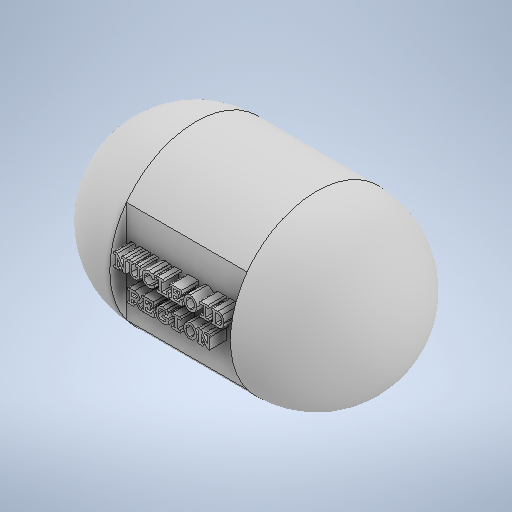
# Autodesk Inventor part: Nucleoid Region
Saved by Autodesk Inventor 2025 (Build 290162000, 162)
## iProperties
Created: 2024-09-07
Part Number: Nucleoid Region
Material: Generic
Document SubType Name: Modeling
Designer: kellst1
Density: 1 g/cm^3
Appearance: Default
Author: kellst1
Autodesk Inventor part; units mm, degrees
ref_plane "YZ Plane" through (0, 0, 0) normal (1, 0, 0) x (0, 1, 0)
ref_plane "XZ Plane" through (0, 0, 0) normal (0, 1, 0) x (-1, 0, 0)
sketch "Sketch2" plane through (0, 0, 0) normal (1, 0, 0) x (0, 1, 0)
  circle A0 centre (0, 0) radius 25
  dimension "d0" = 50
  constraints: 1 centre point, 1 coincident
  measures "d0" diameter of A0
extrude "Extrusion1" add sketch "Sketch2" along normal blind 35
sketch "Sketch3" plane through (35, 0, 0) normal (1, 0, 0) x (0, 0, -1)
  arc A0 (25, 0) -> (-25, 0) centre (0, 0) ccw
  line L0 (-25, 0) -> (25, 0)
  constraints: 2 end point, 2 point on circle, 1 centre point, 1 coincident, 1 horizontal
revolve "Revolution1" add sketch "Sketch3" angle 180 about axis through (35, 0, 25) along (0, 0, -1)
sketch "Sketch4" plane through (0, 0, 0) normal (-1, 0, 0) x (0, 0, 1)
  circle A0 centre (0, 0) radius 25 projected
  line L0 (20.1665, 14.7754) -> (33.009, 14.7754)
  line L1 (33.009, 14.7754) -> (33.009, -19.9353)
  line L2 (33.009, -19.9353) -> (20.1665, -19.9353)
  line L3 (20.1665, -19.9353) -> (20.1665, 14.7754)
  point P0 (20.1665, -14.7754)
  constraints: 8 end point, 2 parallel, 1 horizontal, 1 perpendicular, 2 other
extrude "Extrusion2" cut sketch "Sketch4" against normal blind 35 contours A0 L3 picked at (21.0481, -3.4098)
ref_plane "Work Plane1" through (17.5, 0, 0) normal (-1, 0, 0) x (0, 0, 1)
mirror "Mirror1" about plane through (17.5, 0, 0) normal (-1, 0, 0) of "Revolution1"
sketch "Sketch8" plane through (35, -14.7754, 20.1665) normal (0, 0, 1) x (1, 0, 0)
  line L0 (-34.9965, 29.6893) -> (-0.1735, 29.6893) construction
  line L1 (-0.1735, 29.6893) -> (-0.1735, 0.1878) construction
  line L2 (-0.1735, 0.1878) -> (-34.9965, 0.1878) construction
  line L3 (-34.9965, 0.1878) -> (-34.9965, 29.6893) construction
  line L4 (-32.6139, 19.1334) -> (-32.6139, 17.0905)
  line L5 (-32.6139, 17.0905) -> (-32.3712, 17.0905)
  spline S0 degree 2 poles (-32.3712, 17.0905) (-32.1172, 17.0905) (-31.908, 16.9037) (-31.908, 16.7506) knots 0 0 0 1 2 2 2
  spline S1 degree 2 poles (-31.908, 16.7506) (-31.908, 16.5975) (-32.1172, 16.4145) (-32.3712, 16.4145) knots 0 0 0 1 2 2 2
  line L6 (-32.3712, 16.4145) -> (-33.2899, 16.4145)
  spline S2 degree 2 poles (-33.2899, 16.4145) (-33.5439, 16.4145) (-33.753, 16.6012) (-33.753, 16.7543) knots 0 0 0 1 2 2 2
  spline S3 degree 2 poles (-33.753, 16.7543) (-33.753, 16.9075) (-33.5439, 17.0905) (-33.2899, 17.0905) knots 0 0 0 1 2 2 2
  line L7 (-33.2899, 17.0905) -> (-33.2899, 19.7385)
  line L8 (-33.2899, 19.7385) -> (-33.3945, 19.7385)
  spline S4 degree 2 poles (-33.3945, 19.7385) (-33.6485, 19.7385) (-33.8576, 19.9252) (-33.8576, 20.0783) knots 0 0 0 1 2 2 2
  spline S5 degree 2 poles (-33.8576, 20.0783) (-33.8576, 20.2277) (-33.6485, 20.4145) (-33.3945, 20.4145) knots 0 0 0 1 2 2 2
  line L9 (-33.3945, 20.4145) -> (-32.6177, 20.4107)
  line L10 (-32.6177, 20.4107) -> (-30.881, 17.6992)
  line L11 (-30.881, 17.6992) -> (-30.881, 19.7385)
  line L12 (-30.881, 19.7385) -> (-31.1237, 19.7385)
  spline S6 degree 2 poles (-31.1237, 19.7385) (-31.3777, 19.7385) (-31.5868, 19.9252) (-31.5868, 20.0783) knots 0 0 0 1 2 2 2
  spline S7 degree 2 poles (-31.5868, 20.0783) (-31.5868, 20.2277) (-31.3777, 20.4145) (-31.1237, 20.4145) knots 0 0 0 1 2 2 2
  line L13 (-31.1237, 20.4145) -> (-30.205, 20.4107)
  spline S8 degree 2 poles (-30.205, 20.4107) (-29.951, 20.4107) (-29.7418, 20.2277) (-29.7418, 20.0746) knots 0 0 0 1 2 2 2
  spline S9 degree 2 poles (-29.7418, 20.0746) (-29.7418, 19.9215) (-29.951, 19.7347) (-30.205, 19.7347) knots 0 0 0 1 2 2 2
  line L14 (-30.205, 19.7347) -> (-30.205, 16.4145)
  line L15 (-30.205, 16.4145) -> (-30.8698, 16.4145)
  line L16 (-30.8698, 16.4145) -> (-32.6139, 19.1334)
  line L17 (-26.1713, 19.7347) -> (-26.1713, 17.8188)
  spline S10 degree 2 poles (-26.1713, 17.8188) (-26.1713, 17.195) (-27.0714, 16.3174) (-27.7026, 16.3174) knots 0 0 0 1 2 2 2
  spline S11 degree 2 poles (-27.7026, 16.3174) (-28.0164, 16.3174) (-28.5654, 16.5377) (-29.0061, 16.9672) (-29.2488, 17.4303) (-29.2488, 17.8188) knots 0 0 0 1 2 3 4 4 4
  line L18 (-29.2488, 17.8188) -> (-29.2488, 19.7347)
  spline S12 degree 2 poles (-29.2488, 19.7347) (-29.5028, 19.7347) (-29.712, 19.9215) (-29.712, 20.0746) knots 0 0 0 1 2 2 2
  spline S13 degree 2 poles (-29.712, 20.0746) (-29.712, 20.2277) (-29.5028, 20.4107) (-29.2488, 20.4107) knots 0 0 0 1 2 2 2
  line L19 (-29.2488, 20.4107) -> (-28.3301, 20.4145)
  spline S14 degree 2 poles (-28.3301, 20.4145) (-28.1097, 20.4145) (-27.9006, 20.2277) (-27.9006, 20.0783) knots 0 0 0 1 2 2 2
  spline S15 degree 2 poles (-27.9006, 20.0783) (-27.9006, 19.9252) (-28.1097, 19.7385) (-28.3301, 19.7385) knots 0 0 0 1 2 2 2
  line L20 (-28.3301, 19.7385) -> (-28.5728, 19.7385)
  line L21 (-28.5728, 19.7385) -> (-28.5728, 17.7627)
  spline S16 degree 2 poles (-28.5728, 17.7627) (-28.5728, 17.4602) (-28.0686, 16.9934) (-27.7138, 16.9934) knots 0 0 0 1 2 2 2
  spline S17 degree 2 poles (-27.7138, 16.9934) (-27.4748, 16.9934) (-27.0602, 17.2174) (-26.9295, 17.4341) knots 0 0 0 1 2 2 2
  spline S18 degree 2 poles (-26.9295, 17.4341) (-26.8474, 17.5685) (-26.8474, 17.7627) knots 0 0 0 1 1 1
  line L22 (-26.8474, 17.7627) -> (-26.8474, 19.7385)
  line L23 (-26.8474, 19.7385) -> (-27.0901, 19.7385)
  spline S19 degree 2 poles (-27.0901, 19.7385) (-27.3105, 19.7385) (-27.5196, 19.9252) (-27.5196, 20.0783) knots 0 0 0 1 2 2 2
  spline S20 degree 2 poles (-27.5196, 20.0783) (-27.5196, 20.2277) (-27.3105, 20.4145) (-27.0901, 20.4145) knots 0 0 0 1 2 2 2
  line L24 (-27.0901, 20.4145) -> (-26.1713, 20.4107)
  spline S21 degree 2 poles (-26.1713, 20.4107) (-25.9174, 20.4107) (-25.7082, 20.2277) (-25.7082, 20.0746) knots 0 0 0 1 2 2 2
  spline S22 degree 2 poles (-25.7082, 20.0746) (-25.7082, 19.9215) (-25.9174, 19.7347) (-26.1713, 19.7347) knots 0 0 0 1 2 2 2
  spline S23 degree 2 poles (-22.6046, 20.2389) (-22.5411, 20.3248) (-22.3917, 20.4107) (-22.3058, 20.4107) knots 0 0 0 1 2 2 2
  spline S24 degree 2 poles (-22.3058, 20.4107) (-22.1564, 20.4107) (-21.9697, 20.2053) (-21.9697, 19.9625) knots 0 0 0 1 2 2 2
  line L25 (-21.9697, 19.9625) -> (-21.9697, 19.3874)
  spline S25 degree 2 poles (-21.9697, 19.3874) (-21.9697, 19.1446) (-22.1564, 18.9355) (-22.3058, 18.9355) knots 0 0 0 1 2 2 2
  spline S26 degree 2 poles (-22.3058, 18.9355) (-22.4403, 18.9355) (-22.5224, 19.0102) knots 0 0 0 1 1 1
  spline S27 degree 2 poles (-22.5224, 19.0102) (-22.6046, 19.0886) (-22.6457, 19.294) knots 0 0 0 1 1 1
  spline S28 degree 2 poles (-22.6457, 19.294) (-22.6681, 19.4322) (-22.739, 19.5106) knots 0 0 0 1 1 1
  spline S29 degree 2 poles (-22.739, 19.5106) (-22.8735, 19.6563) (-23.359, 19.8356) (-23.6018, 19.8356) knots 0 0 0 1 2 2 2
  spline S30 degree 2 poles (-23.6018, 19.8356) (-23.9043, 19.8356) (-24.4122, 19.5704) (-24.8007, 18.9803) (-24.8007, 18.5695) knots 0 0 0 1 2 3 3 3
  line L26 (-24.8007, 18.5695) -> (-24.8007, 18.1325)
  spline S31 degree 2 poles (-24.8007, 18.1325) (-24.8007, 17.647) (-24.0911, 16.9934) (-23.4636, 16.9934) knots 0 0 0 1 2 2 2
  spline S32 degree 2 poles (-23.4636, 16.9934) (-23.0864, 16.9934) (-22.8287, 17.0942) knots 0 0 0 1 1 1
  spline S33 degree 2 poles (-22.8287, 17.0942) (-22.6756, 17.154) (-22.5037, 17.3295) knots 0 0 0 1 1 1
  spline S34 degree 2 poles (-22.5037, 17.3295) (-22.3992, 17.4341) (-22.2797, 17.4976) (-22.205, 17.4976) knots 0 0 0 1 2 2 2
  spline S35 degree 2 poles (-22.205, 17.4976) (-22.0705, 17.4976) (-21.8651, 17.2921) (-21.8651, 17.154) knots 0 0 0 1 2 2 2
  spline S36 degree 2 poles (-21.8651, 17.154) (-21.8651, 17.0158) (-22.0033, 16.8589) knots 0 0 0 1 1 1
  spline S37 degree 2 poles (-22.0033, 16.8589) (-22.205, 16.6273) (-22.5224, 16.4966) knots 0 0 0 1 1 1
  spline S38 degree 2 poles (-22.5224, 16.4966) (-22.9445, 16.3174) (-23.4599, 16.3174) knots 0 0 0 1 1 1
  spline S39 degree 2 poles (-23.4599, 16.3174) (-24.0612, 16.3174) (-24.5392, 16.5639) knots 0 0 0 1 1 1
  spline S40 degree 2 poles (-24.5392, 16.5639) (-24.9314, 16.7618) (-25.4767, 17.6171) (-25.4767, 18.1213) knots 0 0 0 1 2 2 2
  line L27 (-25.4767, 18.1213) -> (-25.4767, 18.5769)
  spline S41 degree 2 poles (-25.4767, 18.5769) (-25.4767, 19.1035) (-24.9874, 20.0186) (-24.1172, 20.5116) (-23.6279, 20.5116) knots 0 0 0 1 2 3 3 3
  spline S42 degree 2 poles (-23.6279, 20.5116) (-23.3366, 20.5116) (-22.8249, 20.3771) (-22.6046, 20.2389) knots 0 0 0 1 2 2 2
  line L28 (-19.8931, 19.7347) -> (-19.8931, 17.0905)
  line L29 (-19.8931, 17.0905) -> (-18.4365, 17.0905)
  line L30 (-18.4365, 17.0905) -> (-18.4365, 17.7291)
  spline S43 degree 2 poles (-18.4365, 17.7291) (-18.4365, 17.9831) (-18.2498, 18.1922) (-18.0967, 18.1922) knots 0 0 0 1 2 2 2
  spline S44 degree 2 poles (-18.0967, 18.1922) (-17.9435, 18.1922) (-17.7605, 17.9831) (-17.7605, 17.7291) knots 0 0 0 1 2 2 2
  line L31 (-17.7605, 17.7291) -> (-17.7605, 16.4145)
  line L32 (-17.7605, 16.4145) -> (-20.9613, 16.4145)
  spline S45 degree 2 poles (-20.9613, 16.4145) (-21.2152, 16.4145) (-21.4244, 16.6012) (-21.4244, 16.7543) knots 0 0 0 1 2 2 2
  spline S46 degree 2 poles (-21.4244, 16.7543) (-21.4244, 16.9075) (-21.2152, 17.0905) (-20.9613, 17.0905) knots 0 0 0 1 2 2 2
  line L33 (-20.9613, 17.0905) -> (-20.5691, 17.0905)
  line L34 (-20.5691, 17.0905) -> (-20.5691, 19.7385)
  line L35 (-20.5691, 19.7385) -> (-20.9613, 19.7385)
  spline S47 degree 2 poles (-20.9613, 19.7385) (-21.2152, 19.7385) (-21.4244, 19.9252) (-21.4244, 20.0783) knots 0 0 0 1 2 2 2
  spline S48 degree 2 poles (-21.4244, 20.0783) (-21.4244, 20.2277) (-21.2152, 20.4145) (-20.9613, 20.4145) knots 0 0 0 1 2 2 2
  line L36 (-20.9613, 20.4145) -> (-19.4972, 20.4107)
  spline S49 degree 2 poles (-19.4972, 20.4107) (-19.2432, 20.4107) (-19.0341, 20.2277) (-19.0341, 20.0746) knots 0 0 0 1 2 2 2
  spline S50 degree 2 poles (-19.0341, 20.0746) (-19.0341, 19.9215) (-19.2432, 19.7347) (-19.4972, 19.7347) knots 0 0 0 1 2 2 2
  line L37 (-19.4972, 19.7347) -> (-19.8931, 19.7347)
  line L38 (-16.2516, 18.0839) -> (-16.2516, 17.0905)
  line L39 (-16.2516, 17.0905) -> (-14.5262, 17.0905)
  line L40 (-14.5262, 17.0905) -> (-14.5262, 17.4565)
  spline S51 degree 2 poles (-14.5262, 17.4565) (-14.5262, 17.7104) (-14.3394, 17.9196) (-14.1863, 17.9196) knots 0 0 0 1 2 2 2
  spline S52 degree 2 poles (-14.1863, 17.9196) (-14.0332, 17.9196) (-13.8502, 17.7104) (-13.8502, 17.4565) knots 0 0 0 1 2 2 2
  line L41 (-13.8502, 17.4565) -> (-13.8502, 16.4145)
  line L42 (-13.8502, 16.4145) -> (-17.0322, 16.4145)
  spline S53 degree 2 poles (-17.0322, 16.4145) (-17.2862, 16.4145) (-17.4953, 16.6012) (-17.4953, 16.7543) knots 0 0 0 1 2 2 2
  spline S54 degree 2 poles (-17.4953, 16.7543) (-17.4953, 16.9075) (-17.2862, 17.0905) (-17.0322, 17.0905) knots 0 0 0 1 2 2 2
  line L43 (-17.0322, 17.0905) -> (-16.9277, 17.0905)
  line L44 (-16.9277, 17.0905) -> (-16.9277, 19.7385)
  line L45 (-16.9277, 19.7385) -> (-17.0322, 19.7385)
  spline S55 degree 2 poles (-17.0322, 19.7385) (-17.2862, 19.7385) (-17.4953, 19.9252) (-17.4953, 20.0783) knots 0 0 0 1 2 2 2
  spline S56 degree 2 poles (-17.4953, 20.0783) (-17.4953, 20.2277) (-17.2862, 20.4145) (-17.0322, 20.4145) knots 0 0 0 1 2 2 2
  line L46 (-17.0322, 20.4145) -> (-13.9995, 20.4107)
  line L47 (-13.9995, 20.4107) -> (-13.9995, 19.3874)
  spline S57 degree 2 poles (-13.9995, 19.3874) (-13.9995, 19.1334) (-14.1826, 18.9243) (-14.3357, 18.9243) knots 0 0 0 1 2 2 2
  spline S58 degree 2 poles (-14.3357, 18.9243) (-14.4888, 18.9243) (-14.6756, 19.1334) (-14.6756, 19.3874) knots 0 0 0 1 2 2 2
  line L48 (-14.6756, 19.3874) -> (-14.6756, 19.7385)
  line L49 (-14.6756, 19.7385) -> (-16.2516, 19.7385)
  line L50 (-16.2516, 19.7385) -> (-16.2516, 18.7599)
  line L51 (-16.2516, 18.7599) -> (-15.6578, 18.7599)
  spline S59 degree 2 poles (-15.6578, 18.7599) (-15.6578, 19.0139) (-15.5981, 19.0811) knots 0 0 0 1 1 1
  spline S60 degree 2 poles (-15.5981, 19.0811) (-15.4711, 19.2231) (-15.3179, 19.2231) knots 0 0 0 1 1 1
  spline S61 degree 2 poles (-15.3179, 19.2231) (-15.1648, 19.2231) (-14.9818, 19.0139) (-14.9818, 18.7599) knots 0 0 0 1 2 2 2
  line L52 (-14.9818, 18.7599) -> (-14.9818, 18.0839)
  spline S62 degree 2 poles (-14.9818, 18.0839) (-14.9818, 17.83) (-15.0416, 17.759) knots 0 0 0 1 1 1
  spline S63 degree 2 poles (-15.0416, 17.759) (-15.1648, 17.6208) (-15.3179, 17.6208) knots 0 0 0 1 1 1
  spline S64 degree 2 poles (-15.3179, 17.6208) (-15.4711, 17.6208) (-15.5981, 17.7627) knots 0 0 0 1 1 1
  spline S65 degree 2 poles (-15.5981, 17.7627) (-15.6578, 17.83) (-15.6578, 18.0839) knots 0 0 0 1 1 1
  line L53 (-15.6578, 18.0839) -> (-16.2516, 18.0839)
  spline S66 degree 2 poles (-9.6111, 18.4126) (-9.6111, 17.5125) (-10.7577, 16.3174) (-11.5084, 16.3174) knots 0 0 0 1 2 2 2
  spline S67 degree 2 poles (-11.5084, 16.3174) (-12.1844, 16.3174) (-12.7297, 16.8141) knots 0 0 0 1 1 1
  spline S68 degree 2 poles (-12.7297, 16.8141) (-13.402, 17.4303) (-13.402, 18.4126) knots 0 0 0 1 1 1
  spline S69 degree 2 poles (-13.402, 18.4126) (-13.402, 19.3949) (-12.7297, 20.0148) knots 0 0 0 1 1 1
  spline S70 degree 2 poles (-12.7297, 20.0148) (-12.1844, 20.5116) (-11.5084, 20.5116) knots 0 0 0 1 1 1
  spline S71 degree 2 poles (-11.5084, 20.5116) (-10.7577, 20.5116) (-9.6111, 19.3164) (-9.6111, 18.4126) knots 0 0 0 1 2 2 2
  spline S72 degree 2 poles (-10.2871, 18.4126) (-10.2871, 19.0288) (-11.0341, 19.8356) (-11.5084, 19.8356) knots 0 0 0 1 2 2 2
  spline S73 degree 2 poles (-11.5084, 19.8356) (-11.979, 19.8356) (-12.726, 19.0251) (-12.726, 18.4126) knots 0 0 0 1 2 2 2
  spline S74 degree 2 poles (-12.726, 18.4126) (-12.726, 17.8001) (-11.979, 16.9934) (-11.5084, 16.9934) knots 0 0 0 1 2 2 2
  spline S75 degree 2 poles (-11.5084, 16.9934) (-11.0341, 16.9934) (-10.2871, 17.7963) (-10.2871, 18.4126) knots 0 0 0 1 2 2 2
  line L54 (-7.1163, 19.7347) -> (-7.1163, 17.0905)
  line L55 (-7.1163, 17.0905) -> (-6.4328, 17.0905)
  spline S76 degree 2 poles (-6.4328, 17.0905) (-6.1788, 17.0905) (-5.9697, 16.9037) (-5.9697, 16.7506) knots 0 0 0 1 2 2 2
  spline S77 degree 2 poles (-5.9697, 16.7506) (-5.9697, 16.5975) (-6.1788, 16.4145) (-6.4328, 16.4145) knots 0 0 0 1 2 2 2
  line L56 (-6.4328, 16.4145) -> (-8.4757, 16.4145)
  spline S78 degree 2 poles (-8.4757, 16.4145) (-8.7297, 16.4145) (-8.9389, 16.6012) (-8.9389, 16.7543) knots 0 0 0 1 2 2 2
  spline S79 degree 2 poles (-8.9389, 16.7543) (-8.9389, 16.9075) (-8.7297, 17.0905) (-8.4757, 17.0905) knots 0 0 0 1 2 2 2
  line L57 (-8.4757, 17.0905) -> (-7.7923, 17.0905)
  line L58 (-7.7923, 17.0905) -> (-7.7923, 19.7385)
  line L59 (-7.7923, 19.7385) -> (-8.4757, 19.7385)
  spline S80 degree 2 poles (-8.4757, 19.7385) (-8.7297, 19.7385) (-8.9389, 19.9252) (-8.9389, 20.0783) knots 0 0 0 1 2 2 2
  spline S81 degree 2 poles (-8.9389, 20.0783) (-8.9389, 20.2277) (-8.7297, 20.4145) (-8.4757, 20.4145) knots 0 0 0 1 2 2 2
  line L60 (-8.4757, 20.4145) -> (-6.4328, 20.4107)
  spline S82 degree 2 poles (-6.4328, 20.4107) (-6.1788, 20.4107) (-5.9697, 20.2277) (-5.9697, 20.0746) knots 0 0 0 1 2 2 2
  spline S83 degree 2 poles (-5.9697, 20.0746) (-5.9697, 19.9215) (-6.1788, 19.7347) (-6.4328, 19.7347) knots 0 0 0 1 2 2 2
  line L61 (-6.4328, 19.7347) -> (-7.1163, 19.7347)
  line L62 (-4.9127, 17.0905) -> (-4.9127, 19.7385)
  spline S84 degree 2 poles (-4.9127, 19.7385) (-5.1667, 19.7385) (-5.3758, 19.9252) (-5.3758, 20.0783) knots 0 0 0 1 2 2 2
  spline S85 degree 2 poles (-5.3758, 20.0783) (-5.3758, 20.2277) (-5.1667, 20.4145) (-4.9127, 20.4145) knots 0 0 0 1 2 2 2
  line L63 (-4.9127, 20.4145) -> (-3.486, 20.4107)
  spline S86 degree 2 poles (-3.486, 20.4107) (-3.1536, 20.4107) (-2.515, 20.168) (-2.3245, 19.9775) knots 0 0 0 1 2 2 2
  spline S87 degree 2 poles (-2.3245, 19.9775) (-2.1751, 19.8356) (-1.8614, 19.3426) (-1.7008, 18.8533) (-1.7008, 18.5022) knots 0 0 0 1 2 3 3 3
  line L64 (-1.7008, 18.5022) -> (-1.7008, 18.1773)
  spline S88 degree 2 poles (-1.7008, 18.1773) (-1.7008, 17.7515) (-1.9921, 17.0867) (-2.4701, 16.6684) (-2.6793, 16.5713) knots 0 0 0 1 2 3 3 3
  spline S89 degree 2 poles (-2.6793, 16.5713) (-3.0117, 16.4145) (-3.542, 16.4145) knots 0 0 0 1 1 1
  line L65 (-3.542, 16.4145) -> (-4.9127, 16.4145)
  spline S90 degree 2 poles (-4.9127, 16.4145) (-5.1667, 16.4145) (-5.3758, 16.6012) (-5.3758, 16.7543) knots 0 0 0 1 2 2 2
  spline S91 degree 2 poles (-5.3758, 16.7543) (-5.3758, 16.9075) (-5.1667, 17.0905) (-4.9127, 17.0905) knots 0 0 0 1 2 2 2
  line L66 (-4.2367, 17.0905) -> (-3.5196, 17.0905)
  spline S92 degree 2 poles (-3.5196, 17.0905) (-3.1163, 17.0905) (-2.9146, 17.2062) knots 0 0 0 1 1 1
  spline S93 degree 2 poles (-2.9146, 17.2062) (-2.6457, 17.3594) (-2.3768, 17.8262) (-2.3768, 18.1997) knots 0 0 0 1 2 2 2
  line L67 (-2.3768, 18.1997) -> (-2.3768, 18.5209)
  spline S94 degree 2 poles (-2.3768, 18.5209) (-2.3768, 18.8421) (-2.5, 19.0811) knots 0 0 0 1 1 1
  spline S95 degree 2 poles (-2.5, 19.0811) (-2.6905, 19.4583) (-3.1685, 19.7385) (-3.5271, 19.7385) knots 0 0 0 1 2 2 2
  line L68 (-3.5271, 19.7385) -> (-4.2367, 19.7385)
  line L69 (-4.2367, 19.7385) -> (-4.2367, 17.0905)
  line L70 (-28.444, 10.9902) -> (-28.444, 10.1387)
  line L71 (-28.444, 10.1387) -> (-28.2012, 10.1387)
  spline S96 degree 2 poles (-28.2012, 10.1387) (-27.9473, 10.1387) (-27.7381, 9.9519) (-27.7381, 9.7988) knots 0 0 0 1 2 2 2
  spline S97 degree 2 poles (-27.7381, 9.7988) (-27.7381, 9.6457) (-27.9473, 9.4627) (-28.2012, 9.4627) knots 0 0 0 1 2 2 2
  line L72 (-28.2012, 9.4627) -> (-29.2246, 9.4627)
  spline S98 degree 2 poles (-29.2246, 9.4627) (-29.4785, 9.4627) (-29.6877, 9.6494) (-29.6877, 9.8026) knots 0 0 0 1 2 2 2
  spline S99 degree 2 poles (-29.6877, 9.8026) (-29.6877, 9.9557) (-29.4785, 10.1387) (-29.2246, 10.1387) knots 0 0 0 1 2 2 2
  line L73 (-29.2246, 10.1387) -> (-29.12, 10.1387)
  line L74 (-29.12, 10.1387) -> (-29.12, 12.7867)
  line L75 (-29.12, 12.7867) -> (-29.2246, 12.7867)
  spline S100 degree 2 poles (-29.2246, 12.7867) (-29.4785, 12.7867) (-29.6877, 12.9734) (-29.6877, 13.1265) knots 0 0 0 1 2 2 2
  spline S101 degree 2 poles (-29.6877, 13.1265) (-29.6877, 13.2759) (-29.4785, 13.4627) (-29.2246, 13.4627) knots 0 0 0 1 2 2 2
  line L76 (-29.2246, 13.4627) -> (-27.6933, 13.4589)
  spline S102 degree 2 poles (-27.6933, 13.4589) (-26.9799, 13.4589) (-26.1919, 12.7493) (-26.1919, 12.2414) knots 0 0 0 1 2 2 2
  spline S103 degree 2 poles (-26.1919, 12.2414) (-26.1919, 11.9277) (-26.5616, 11.4085) (-26.9351, 11.2068) knots 0 0 0 1 2 2 2
  spline S104 degree 2 poles (-26.9351, 11.2068) (-26.7185, 11.0201) (-26.4757, 10.7251) knots 0 0 0 1 1 1
  spline S105 degree 2 poles (-26.4757, 10.7251) (-26.3226, 10.5383) (-26.0649, 10.1387) knots 0 0 0 1 1 1
  spline S106 degree 2 poles (-26.0649, 10.1387) (-25.8109, 10.1387) (-25.7362, 10.0752) knots 0 0 0 1 1 1
  spline S107 degree 2 poles (-25.7362, 10.0752) (-25.6018, 9.9519) (-25.6018, 9.7988) knots 0 0 0 1 1 1
  spline S108 degree 2 poles (-25.6018, 9.7988) (-25.6018, 9.6457) (-25.8109, 9.4627) (-26.0649, 9.4627) knots 0 0 0 1 2 2 2
  line L77 (-26.0649, 9.4627) -> (-26.4122, 9.4627)
  spline S109 degree 2 poles (-26.4122, 9.4627) (-27.2339, 10.7325) (-27.7755, 10.9902) knots 0 0 0 1 1 1
  line L78 (-27.7755, 10.9902) -> (-28.444, 10.9902)
  line L79 (-28.444, 11.6662) -> (-27.9174, 11.6662)
  spline S110 degree 2 poles (-27.9174, 11.6662) (-27.6223, 11.6662) (-27.3908, 11.7559) knots 0 0 0 1 1 1
  spline S111 degree 2 poles (-27.3908, 11.7559) (-27.0808, 11.8754) (-26.8679, 12.1368) (-26.8679, 12.2675) knots 0 0 0 1 2 2 2
  spline S112 degree 2 poles (-26.8679, 12.2675) (-26.8679, 12.458) (-27.275, 12.7829) (-27.6709, 12.7829) knots 0 0 0 1 2 2 2
  line L80 (-27.6709, 12.7829) -> (-28.444, 12.7867)
  line L81 (-28.444, 12.7867) -> (-28.444, 11.6662)
  line L82 (-24.388, 11.1321) -> (-24.388, 10.1387)
  line L83 (-24.388, 10.1387) -> (-22.6625, 10.1387)
  line L84 (-22.6625, 10.1387) -> (-22.6625, 10.5047)
  spline S113 degree 2 poles (-22.6625, 10.5047) (-22.6625, 10.7587) (-22.4757, 10.9678) (-22.3226, 10.9678) knots 0 0 0 1 2 2 2
  spline S114 degree 2 poles (-22.3226, 10.9678) (-22.1695, 10.9678) (-21.9865, 10.7587) (-21.9865, 10.5047) knots 0 0 0 1 2 2 2
  line L85 (-21.9865, 10.5047) -> (-21.9865, 9.4627)
  line L86 (-21.9865, 9.4627) -> (-25.1685, 9.4627)
  spline S115 degree 2 poles (-25.1685, 9.4627) (-25.4225, 9.4627) (-25.6317, 9.6494) (-25.6317, 9.8026) knots 0 0 0 1 2 2 2
  spline S116 degree 2 poles (-25.6317, 9.8026) (-25.6317, 9.9557) (-25.4225, 10.1387) (-25.1685, 10.1387) knots 0 0 0 1 2 2 2
  line L87 (-25.1685, 10.1387) -> (-25.064, 10.1387)
  line L88 (-25.064, 10.1387) -> (-25.064, 12.7867)
  line L89 (-25.064, 12.7867) -> (-25.1685, 12.7867)
  spline S117 degree 2 poles (-25.1685, 12.7867) (-25.4225, 12.7867) (-25.6317, 12.9734) (-25.6317, 13.1265) knots 0 0 0 1 2 2 2
  spline S118 degree 2 poles (-25.6317, 13.1265) (-25.6317, 13.2759) (-25.4225, 13.4627) (-25.1685, 13.4627) knots 0 0 0 1 2 2 2
  line L90 (-25.1685, 13.4627) -> (-22.1359, 13.4589)
  line L91 (-22.1359, 13.4589) -> (-22.1359, 12.4356)
  spline S119 degree 2 poles (-22.1359, 12.4356) (-22.1359, 12.1816) (-22.3189, 11.9725) (-22.472, 11.9725) knots 0 0 0 1 2 2 2
  spline S120 degree 2 poles (-22.472, 11.9725) (-22.6251, 11.9725) (-22.8119, 12.1816) (-22.8119, 12.4356) knots 0 0 0 1 2 2 2
  line L92 (-22.8119, 12.4356) -> (-22.8119, 12.7867)
  line L93 (-22.8119, 12.7867) -> (-24.388, 12.7867)
  line L94 (-24.388, 12.7867) -> (-24.388, 11.8082)
  line L95 (-24.388, 11.8082) -> (-23.7941, 11.8082)
  spline S121 degree 2 poles (-23.7941, 11.8082) (-23.7941, 12.0621) (-23.7344, 12.1293) knots 0 0 0 1 1 1
  spline S122 degree 2 poles (-23.7344, 12.1293) (-23.6074, 12.2713) (-23.4543, 12.2713) knots 0 0 0 1 1 1
  spline S123 degree 2 poles (-23.4543, 12.2713) (-23.3011, 12.2713) (-23.1181, 12.0621) (-23.1181, 11.8082) knots 0 0 0 1 2 2 2
  line L96 (-23.1181, 11.8082) -> (-23.1181, 11.1321)
  spline S124 degree 2 poles (-23.1181, 11.1321) (-23.1181, 10.8782) (-23.1779, 10.8072) knots 0 0 0 1 1 1
  spline S125 degree 2 poles (-23.1779, 10.8072) (-23.3011, 10.669) (-23.4543, 10.669) knots 0 0 0 1 1 1
  spline S126 degree 2 poles (-23.4543, 10.669) (-23.6074, 10.669) (-23.7344, 10.811) knots 0 0 0 1 1 1
  spline S127 degree 2 poles (-23.7344, 10.811) (-23.7941, 10.8782) (-23.7941, 11.1321) knots 0 0 0 1 1 1
  line L97 (-23.7941, 11.1321) -> (-24.388, 11.1321)
  line L98 (-17.9379, 10.6952) -> (-17.9379, 9.7951)
  spline S128 degree 2 poles (-17.9379, 9.7951) (-18.3973, 9.5448) (-19.0397, 9.3656) (-19.4132, 9.3656) knots 0 0 0 1 2 2 2
  spline S129 degree 2 poles (-19.4132, 9.3656) (-19.9323, 9.3656) (-20.373, 9.5187) knots 0 0 0 1 1 1
  spline S130 degree 2 poles (-20.373, 9.5187) (-20.7204, 9.6382) (-21.12, 10.0005) (-21.4561, 10.7101) (-21.4561, 11.1471) knots 0 0 0 1 2 3 3 3
  line L99 (-21.4561, 11.1471) -> (-21.4561, 11.6364)
  spline S131 degree 2 poles (-21.4561, 11.6364) (-21.4561, 12.3124) (-21.0453, 12.8427) knots 0 0 0 1 1 1
  spline S132 degree 2 poles (-21.0453, 12.8427) (-20.4888, 13.5598) (-19.5364, 13.5598) knots 0 0 0 1 1 1
  spline S133 degree 2 poles (-19.5364, 13.5598) (-19.2601, 13.5598) (-18.7596, 13.4477) (-18.5355, 13.3357) knots 0 0 0 1 2 2 2
  spline S134 degree 2 poles (-18.5355, 13.3357) (-18.401, 13.4589) (-18.2703, 13.4589) knots 0 0 0 1 1 1
  spline S135 degree 2 poles (-18.2703, 13.4589) (-18.1209, 13.4589) (-17.9379, 13.2535) (-17.9379, 13.0108) knots 0 0 0 1 2 2 2
  line L100 (-17.9379, 13.0108) -> (-17.9379, 12.5738)
  spline S136 degree 2 poles (-17.9379, 12.5738) (-17.9379, 12.331) (-18.1247, 12.1219) (-18.2741, 12.1219) knots 0 0 0 1 2 2 2
  spline S137 degree 2 poles (-18.2741, 12.1219) (-18.3936, 12.1219) (-18.4795, 12.1928) knots 0 0 0 1 1 1
  spline S138 degree 2 poles (-18.4795, 12.1928) (-18.5467, 12.2451) (-18.6363, 12.5813) (-18.6924, 12.641) knots 0 0 0 1 2 2 2
  spline S139 degree 2 poles (-18.6924, 12.641) (-18.7783, 12.7344) (-19.2302, 12.8838) (-19.514, 12.8838) knots 0 0 0 1 2 2 2
  spline S140 degree 2 poles (-19.514, 12.8838) (-19.9136, 12.8838) (-20.2124, 12.7195) knots 0 0 0 1 1 1
  spline S141 degree 2 poles (-20.2124, 12.7195) (-20.4253, 12.5962) (-20.7801, 11.9912) (-20.7801, 11.6364) knots 0 0 0 1 2 2 2
  line L101 (-20.7801, 11.6364) -> (-20.7801, 11.1471)
  spline S142 degree 2 poles (-20.7801, 11.1471) (-20.7801, 10.6055) (-20.1489, 10.0416) (-19.4617, 10.0416) knots 0 0 0 1 2 2 2
  spline S143 degree 2 poles (-19.4617, 10.0416) (-18.9986, 10.0416) (-18.6139, 10.2134) knots 0 0 0 1 1 1
  line L102 (-18.6139, 10.2134) -> (-18.6139, 10.6989)
  line L103 (-18.6139, 10.6989) -> (-19.3049, 10.6989)
  spline S144 degree 2 poles (-19.3049, 10.6989) (-19.5588, 10.6989) (-19.768, 10.8857) (-19.768, 11.0388) knots 0 0 0 1 2 2 2
  spline S145 degree 2 poles (-19.768, 11.0388) (-19.768, 11.1882) (-19.5588, 11.3749) (-19.3049, 11.3749) knots 0 0 0 1 2 2 2
  line L104 (-19.3049, 11.3749) -> (-17.9379, 11.3712)
  spline S146 degree 2 poles (-17.9379, 11.3712) (-17.8109, 11.3712) (-17.6018, 11.1882) (-17.6018, 11.035) knots 0 0 0 1 2 2 2
  spline S147 degree 2 poles (-17.6018, 11.035) (-17.6018, 10.8819) (-17.8109, 10.6952) (-17.9379, 10.6952) knots 0 0 0 1 2 2 2
  line L105 (-15.2526, 12.7829) -> (-15.2526, 10.1387)
  line L106 (-15.2526, 10.1387) -> (-14.5691, 10.1387)
  spline S148 degree 2 poles (-14.5691, 10.1387) (-14.3151, 10.1387) (-14.106, 9.9519) (-14.106, 9.7988) knots 0 0 0 1 2 2 2
  spline S149 degree 2 poles (-14.106, 9.7988) (-14.106, 9.6457) (-14.3151, 9.4627) (-14.5691, 9.4627) knots 0 0 0 1 2 2 2
  line L107 (-14.5691, 9.4627) -> (-16.6121, 9.4627)
  spline S150 degree 2 poles (-16.6121, 9.4627) (-16.866, 9.4627) (-17.0752, 9.6494) (-17.0752, 9.8026) knots 0 0 0 1 2 2 2
  spline S151 degree 2 poles (-17.0752, 9.8026) (-17.0752, 9.9557) (-16.866, 10.1387) (-16.6121, 10.1387) knots 0 0 0 1 2 2 2
  line L108 (-16.6121, 10.1387) -> (-15.9286, 10.1387)
  line L109 (-15.9286, 10.1387) -> (-15.9286, 12.7867)
  line L110 (-15.9286, 12.7867) -> (-16.6121, 12.7867)
  spline S152 degree 2 poles (-16.6121, 12.7867) (-16.866, 12.7867) (-17.0752, 12.9734) (-17.0752, 13.1265) knots 0 0 0 1 2 2 2
  spline S153 degree 2 poles (-17.0752, 13.1265) (-17.0752, 13.2759) (-16.866, 13.4627) (-16.6121, 13.4627) knots 0 0 0 1 2 2 2
  line L111 (-16.6121, 13.4627) -> (-14.5691, 13.4589)
  spline S154 degree 2 poles (-14.5691, 13.4589) (-14.3151, 13.4589) (-14.106, 13.2759) (-14.106, 13.1228) knots 0 0 0 1 2 2 2
  spline S155 degree 2 poles (-14.106, 13.1228) (-14.106, 12.9697) (-14.3151, 12.7829) (-14.5691, 12.7829) knots 0 0 0 1 2 2 2
  line L112 (-14.5691, 12.7829) -> (-15.2526, 12.7829)
  spline S156 degree 2 poles (-9.6429, 11.4608) (-9.6429, 10.5607) (-10.7895, 9.3656) (-11.5402, 9.3656) knots 0 0 0 1 2 2 2
  spline S157 degree 2 poles (-11.5402, 9.3656) (-12.2162, 9.3656) (-12.7615, 9.8623) knots 0 0 0 1 1 1
  spline S158 degree 2 poles (-12.7615, 9.8623) (-13.4337, 10.4786) (-13.4337, 11.4608) knots 0 0 0 1 1 1
  spline S159 degree 2 poles (-13.4337, 11.4608) (-13.4337, 12.4431) (-12.7615, 13.0631) knots 0 0 0 1 1 1
  spline S160 degree 2 poles (-12.7615, 13.0631) (-12.2162, 13.5598) (-11.5402, 13.5598) knots 0 0 0 1 1 1
  spline S161 degree 2 poles (-11.5402, 13.5598) (-10.7895, 13.5598) (-9.6429, 12.3646) (-9.6429, 11.4608) knots 0 0 0 1 2 2 2
  spline S162 degree 2 poles (-10.3189, 11.4608) (-10.3189, 12.0771) (-11.0658, 12.8838) (-11.5402, 12.8838) knots 0 0 0 1 2 2 2
  spline S163 degree 2 poles (-11.5402, 12.8838) (-12.0108, 12.8838) (-12.7577, 12.0733) (-12.7577, 11.4608) knots 0 0 0 1 2 2 2
  spline S164 degree 2 poles (-12.7577, 11.4608) (-12.7577, 10.8483) (-12.0108, 10.0416) (-11.5402, 10.0416) knots 0 0 0 1 2 2 2
  spline S165 degree 2 poles (-11.5402, 10.0416) (-11.0658, 10.0416) (-10.3189, 10.8446) (-10.3189, 11.4608) knots 0 0 0 1 2 2 2
  line L113 (-8.3319, 12.1816) -> (-8.3319, 10.1387)
  line L114 (-8.3319, 10.1387) -> (-8.0892, 10.1387)
  spline S166 degree 2 poles (-8.0892, 10.1387) (-7.8352, 10.1387) (-7.6261, 9.9519) (-7.6261, 9.7988) knots 0 0 0 1 2 2 2
  spline S167 degree 2 poles (-7.6261, 9.7988) (-7.6261, 9.6457) (-7.8352, 9.4627) (-8.0892, 9.4627) knots 0 0 0 1 2 2 2
  line L115 (-8.0892, 9.4627) -> (-9.0079, 9.4627)
  spline S168 degree 2 poles (-9.0079, 9.4627) (-9.2619, 9.4627) (-9.4711, 9.6494) (-9.4711, 9.8026) knots 0 0 0 1 2 2 2
  spline S169 degree 2 poles (-9.4711, 9.8026) (-9.4711, 9.9557) (-9.2619, 10.1387) (-9.0079, 10.1387) knots 0 0 0 1 2 2 2
  line L116 (-9.0079, 10.1387) -> (-9.0079, 12.7867)
  line L117 (-9.0079, 12.7867) -> (-9.1125, 12.7867)
  spline S170 degree 2 poles (-9.1125, 12.7867) (-9.3665, 12.7867) (-9.5756, 12.9734) (-9.5756, 13.1265) knots 0 0 0 1 2 2 2
  spline S171 degree 2 poles (-9.5756, 13.1265) (-9.5756, 13.2759) (-9.3665, 13.4627) (-9.1125, 13.4627) knots 0 0 0 1 2 2 2
  line L118 (-9.1125, 13.4627) -> (-8.3357, 13.4589)
  line L119 (-8.3357, 13.4589) -> (-6.599, 10.7475)
  line L120 (-6.599, 10.7475) -> (-6.599, 12.7867)
  line L121 (-6.599, 12.7867) -> (-6.8417, 12.7867)
  spline S172 degree 2 poles (-6.8417, 12.7867) (-7.0957, 12.7867) (-7.3049, 12.9734) (-7.3049, 13.1265) knots 0 0 0 1 2 2 2
  spline S173 degree 2 poles (-7.3049, 13.1265) (-7.3049, 13.2759) (-7.0957, 13.4627) (-6.8417, 13.4627) knots 0 0 0 1 2 2 2
  line L122 (-6.8417, 13.4627) -> (-5.923, 13.4589)
  spline S174 degree 2 poles (-5.923, 13.4589) (-5.669, 13.4589) (-5.4599, 13.2759) (-5.4599, 13.1228) knots 0 0 0 1 2 2 2
  spline S175 degree 2 poles (-5.4599, 13.1228) (-5.4599, 12.9697) (-5.669, 12.7829) (-5.923, 12.7829) knots 0 0 0 1 2 2 2
  line L123 (-5.923, 12.7829) -> (-5.923, 9.4627)
  line L124 (-5.923, 9.4627) -> (-6.5878, 9.4627)
  line L125 (-6.5878, 9.4627) -> (-8.3319, 12.1816)
  point P0 (-35, 14.7754)
  constraints: 2 other
extrude "Extrusion3" add sketch "Sketch8" along normal blind 5
body "Solid1"
